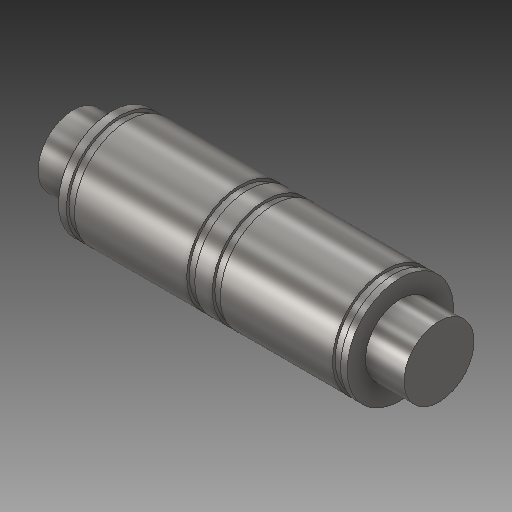
# Autodesk Inventor part: Gearbox Axle 1
Saved by Autodesk Inventor 2019 (Build 230136000, 136)
## iProperties
Created: 2019-11-03
Part Number: Gearbox Axle 1
Material: Stainless Steel
Document SubType Name: Modeling
Designer: admin
Density: 8 g/cm^3
Appearance: Semi-Polished
Author: admin
Autodesk Inventor part; units mm, degrees
ref_plane "YZ Plane" through (0, 0, 0) normal (1, 0, 0) x (0, 1, 0)
ref_plane "XZ Plane" through (0, 0, 0) normal (0, 1, 0) x (-1, 0, 0)
ref_plane "XY Plane" through (0, 0, 0) normal (0, 0, 1) x (1, 0, 0)
sketch "Sketch1" plane through (0, 0, 0) normal (0, 0, 1) x (1, 0, 0)
  line L0 (0, 0) -> (0, 4.8)
  line L1 (0, 4.8) -> (5.3, 4.8)
  line L2 (5.3, 4.8) -> (5.3, 7.3)
  line L3 (5.3, 7.3) -> (6.4, 7.3)
  line L4 (6.4, 7.3) -> (6.4, 6.95)
  line L5 (6.4, 6.95) -> (7.5, 6.95)
  line L6 (7.5, 6.95) -> (7.5, 7.3)
  line L7 (7.5, 7.3) -> (22.9, 7.3)
  line L8 (22.9, 7.3) -> (22.9, 6.95)
  line L9 (22.9, 6.95) -> (24, 6.95)
  line L10 (24, 6.95) -> (24, 7.3)
  line L11 (24, 7.3) -> (26.4, 7.3)
  line L12 (26.4, 7.3) -> (26.4, 6.95)
  line L13 (26.4, 6.95) -> (27.5, 6.95)
  line L14 (27.5, 6.95) -> (27.5, 7.3)
  line L15 (27.5, 7.3) -> (42.9, 7.3)
  line L16 (42.9, 7.3) -> (42.9, 6.95)
  line L17 (42.9, 6.95) -> (44, 6.95)
  line L18 (44, 6.95) -> (44, 7.3)
  line L19 (44, 7.3) -> (44.9, 7.3)
  line L20 (44.9, 7.3) -> (44.9, 4.8)
  line L21 (44.9, 4.8) -> (50.2, 4.8)
  line L22 (50.2, 4.8) -> (50.2, 0)
  line L23 (50.2, 0) -> (0, 0)
  dimension "d0" = 50.2
  dimension "d1" = 5.3
  dimension "d2" = 5.3
  dimension "d3" = 7.3
  dimension "d4" = 1.1
  dimension "d5" = 1.1
  dimension "d6" = 1.1
  dimension "d7" = 1.1
  dimension "d8" = 15.4
  dimension "d9" = 15.4
  dimension "d10" = 4.8
  dimension "d12" = 42.9
  dimension "d13" = 0.35
  dimension "d15" = 7.5
  constraints: 48 end point, 16 point on line, 13 perpendicular, 1 vertical
  measures "d0" distance of L22.end L0.start
  measures "d1" distance of L0.end L1.end
  measures "d2" distance of L20.end L21.end
  measures "d3" distance between parallel lines of L23 L19
  measures "d4" distance of L4.end L5.end
  measures "d5" distance of L8.end L9.end
  measures "d6" distance of L12.end L13.end
  measures "d7" distance of L16.end L17.end
  measures "d8" distance between parallel lines of L16 L14
  measures "d9" distance between parallel lines of L8 L6
  measures "d10" distance between parallel lines of L23 L1
  measures "d12" distance between parallel lines of L0 L16
  measures "d13" distance of L7.end L8.end
  measures "d15" distance from line of L5.end L0
revolve "Revolution1" add sketch "Sketch1" angle 360 about axis through (50.2, 0, 0) along (-1, 0, 0)
body "Solid1"
